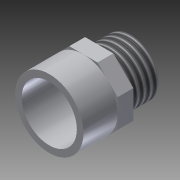
# Autodesk Inventor part: 1 Thread to pipe
Saved by Autodesk Inventor 2013 (Build 170138000, 138)
## iProperties
Created: 2013-06-27
Part Number: 1 Thread to pipe
Material: PVC-Piping
Document SubType Name: Modeling
Designer: Kyle
Density: 1 g/cm^3
Author: Kyle
Autodesk Inventor part; units mm, degrees
ref_plane "YZ Plane" through (0, 0, 0) normal (1, 0, 0) x (0, 1, 0)
ref_plane "XZ Plane" through (0, 0, 0) normal (0, 1, 0) x (-1, 0, 0)
ref_plane "XY Plane" through (0, 0, 0) normal (0, 0, 1) x (1, 0, 0)
sketch "Sketch1" plane through (0, 0, 0) normal (0, 0, 1) x (1, 0, 0)
  circle A0 centre (0, 0) radius 13.335
  circle A1 centre (0, 0) radius 9.525
  dimension "d0" = 26.67
  dimension "d2" = 19.05
  constraints: 2 centre point, 1 coincident
  measures "d0" diameter of A0
  measures "d2" diameter of A1
extrude "Extrusion1" add sketch "Sketch1" along normal blind 15.24
sketch "Sketch2" plane through (0, 0, 15.24) normal (0, 0, 1) x (1, 0, 0)
  circle A0 centre (0, 0) radius 13.335 projected
  line L0 (16.51, -6.8387) -> (6.8387, -16.51)
  line L1 (6.8387, -16.51) -> (-6.8387, -16.51)
  line L2 (-6.8387, -16.51) -> (-16.51, -6.8387)
  line L3 (-16.51, -6.8387) -> (-16.51, 6.8387)
  line L4 (-16.51, 6.8387) -> (-6.8387, 16.51)
  line L5 (-6.8387, 16.51) -> (6.8387, 16.51)
  line L6 (6.8387, 16.51) -> (16.51, 6.8387)
  line L7 (16.51, 6.8387) -> (16.51, -6.8387)
  dimension "d5" = 33.02
  constraints: 16 end point, 1 coincident, 1 vertical, 17 other
  measures "d5" distance between parallel lines of L7 L3
extrude "Extrusion2" add sketch "Sketch2" along normal blind 7.62
sketch "Sketch3" plane through (0, 0, 22.86) normal (0, 0, 1) x (1, 0, 0)
  circle A0 centre (0, 0) radius 13.335 projected
  circle A1 centre (0, 0) radius 16.51
  circle A2 centre (0, 0) radius 13.335
  dimension "d8" = 33.02
  dimension "d10" = 26.67
  constraints: 2 centre point, 1 coincident
  measures "d8" diameter of A1
  measures "d10" diameter of A2
extrude "Extrusion3" add sketch "Sketch3" along normal blind 16.51
thread "Thread1" size "1 1/16-8 UNC" class "2A" standard "ANSI Unified Screw Threads" full length
body "Solid1"
